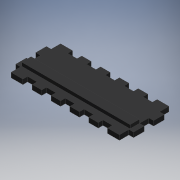
# Autodesk Inventor part: front
Saved by Autodesk Inventor 2019 (Build 230136000, 136)
## iProperties
Created: 2018-06-07
Part Number: front
Material: PBT Plastic Black
Document SubType Name: Modeling
Designer: stra92745
Density: 1.31 g/cm^3
Appearance: Smooth - White
Author: stra92745
Autodesk Inventor part; units mm, degrees
ref_plane "YZ Plane" through (0, 0, 0) normal (1, 0, 0) x (0, 1, 0)
ref_plane "XZ Plane" through (0, 0, 0) normal (0, 1, 0) x (-1, 0, 0)
ref_plane "XY Plane" through (0, 0, 0) normal (0, 0, 1) x (1, 0, 0)
sketch "Sketch1" plane through (0, 0, 0) normal (0, 1, 0) x (-1, 0, 0)
  line L0 (0, 0) -> (-100, 0)
  line L1 (-100, 0) -> (-100, -42)
  line L2 (-100, -42) -> (0, -42)
  line L3 (0, -42) -> (0, 0)
  dimension "d0" = 100
  dimension "d1" = 42
  constraints: 8 end point, 2 parallel, 1 horizontal, 1 perpendicular
  measures "d0" distance of L2.end L1.end
  measures "d1" distance of L1.end L0.end
extrude "Extrusion1" add sketch "Sketch1" along normal blind 4
sketch "Sketch2" plane through (0, 4, 0) normal (0, 1, 0) x (1, 0, 0)
  line L0 (0, 0) -> (100, 0) construction
  line L1 (100, 0) -> (100, 42) construction
  line L2 (100, 42) -> (0, 42) construction
  line L3 (0, 42) -> (0, 0) construction
  line L4 (4, 38) -> (96, 38) construction
  line L5 (96, 38) -> (96, 4) construction
  line L6 (96, 4) -> (4, 4) construction
  line L7 (4, 4) -> (4, 38) construction
  line L8 (100, 42) -> (0, 42) projected
  line L9 (4, 42) -> (4, 34)
  line L10 (4, 34) -> (0, 34)
  line L11 (0, 42) -> (0, 0) projected
  line L12 (0, 34) -> (0, 42)
  line L13 (0, 42) -> (4, 42)
  line L14 (0, 21) -> (100, 21) construction
  line L15 (50, 42) -> (50, 0) construction
  line L16 (0, 0) -> (100, 0) construction
  line L17 (0, 21) -> (0, 25)
  line L18 (4, 25) -> (0, 25)
  line L19 (4, 25) -> (4, 21)
  line L20 (14, 42) -> (14, 38)
  line L21 (14, 38) -> (22, 38)
  line L22 (22, 38) -> (22, 42)
  line L23 (14, 42) -> (22, 42)
  line L24 (30, 42) -> (38, 42)
  line L25 (38, 42) -> (38, 38)
  line L26 (38, 38) -> (30, 38)
  line L27 (30, 38) -> (30, 42)
  line L28 (50, 38) -> (46, 38)
  line L29 (46, 38) -> (46, 42)
  line L30 (46, 42) -> (50, 42)
  line L31 (4, 0) -> (4, 8)
  line L32 (4, 8) -> (0, 8)
  line L33 (0, 8) -> (0, 0)
  line L34 (0, 0) -> (4, 0)
  line L35 (0, 21) -> (0, 17)
  line L36 (4, 17) -> (0, 17)
  line L37 (4, 17) -> (4, 21)
  line L38 (14, 0) -> (14, 4)
  line L39 (14, 4) -> (22, 4)
  line L40 (22, 4) -> (22, 0)
  line L41 (14, 0) -> (22, 0)
  line L42 (30, 0) -> (38, 0)
  line L43 (38, 0) -> (38, 4)
  line L44 (38, 4) -> (30, 4)
  line L45 (30, 4) -> (30, 0)
  line L46 (50, 4) -> (46, 4)
  line L47 (46, 4) -> (46, 0)
  line L48 (46, 0) -> (50, 0)
  line L49 (100, 42) -> (100, 0) construction
  line L50 (96, 4) -> (96, 38) construction
  line L51 (96, 42) -> (96, 34)
  line L52 (96, 34) -> (100, 34)
  line L53 (100, 42) -> (100, 0)
  line L54 (100, 34) -> (100, 42)
  line L55 (100, 42) -> (96, 42)
  line L56 (100, 21) -> (100, 25)
  line L57 (96, 25) -> (100, 25)
  line L58 (96, 25) -> (96, 21)
  line L59 (86, 42) -> (86, 38)
  line L60 (86, 38) -> (78, 38)
  line L61 (78, 38) -> (78, 42)
  line L62 (86, 42) -> (78, 42)
  line L63 (70, 42) -> (62, 42)
  line L64 (62, 42) -> (62, 38)
  line L65 (62, 38) -> (70, 38)
  line L66 (70, 38) -> (70, 42)
  line L67 (50, 38) -> (54, 38)
  line L68 (54, 38) -> (54, 42)
  line L69 (54, 42) -> (50, 42)
  line L70 (70, 4) -> (70, 0)
  line L71 (62, 4) -> (70, 4)
  line L72 (70, 0) -> (62, 0)
  line L73 (62, 0) -> (62, 4)
  line L74 (54, 4) -> (54, 0)
  line L75 (50, 4) -> (54, 4)
  line L76 (54, 0) -> (50, 0)
  line L77 (78, 4) -> (78, 0)
  line L78 (86, 4) -> (78, 4)
  line L79 (86, 0) -> (78, 0)
  line L80 (86, 0) -> (86, 4)
  line L81 (96, 0) -> (96, 8)
  line L82 (100, 0) -> (96, 0)
  line L83 (96, 8) -> (100, 8)
  line L84 (100, 8) -> (100, 0)
  line L85 (96, 17) -> (96, 21)
  line L86 (100, 21) -> (100, 17)
  line L87 (96, 17) -> (100, 17)
  dimension "d4" = 4
  dimension "d5" = 4
  dimension "d7" = 8
  dimension "d8" = 8
  dimension "d10" = 8
  dimension "d11" = 8
  dimension "d13" = 4
  dimension "d14" = 8
  constraints: 162 end point, 49 symmetric about line, 19 point on line, 7 midpoint, 7 perpendicular, 3 collinear, 3 parallel, 1 horizontal, 3 other
  measures "d4" distance between parallel lines of L2 L4
  measures "d5" distance of L18.start L19.end
  measures "d7" distance of L9.start L9.end
  measures "d8" distance of L20.end L21.end
  measures "d10" distance of L25.end L26.end
  measures "d11" distance between parallel lines of L22 L27
  measures "d13" distance of L28.start L28.end
  measures "d14" distance between parallel lines of L25 L29
extrude "Extrusion2" cut sketch "Sketch2" against normal up to surface (4 mm away)
sketch "Sketch3" plane through (0, 4, 0) normal (0, 1, 0) x (1, 0, 0)
  line L0 (4, 25) -> (4, 17) projected
  line L1 (96, 0) -> (96, 8) projected
  line L2 (4, 17) -> (96, 17)
  line L3 (96, 17) -> (96, 9)
  line L4 (96, 9) -> (4, 9)
  line L5 (4, 9) -> (4, 17)
  line L6 (30, 4) -> (38, 4) projected
  point P0 (0, 0)
  dimension "d17" = 5
  dimension "d18" = 8
  constraints: 8 end point, 2 parallel, 2 point on line, 1 horizontal, 1 perpendicular
  measures "d17" distance between parallel lines of L4 L6
  measures "d18" distance between parallel lines of L2 L4
extrude "Extrusion3" add sketch "Sketch3" along normal blind 3
body "Solid1"
